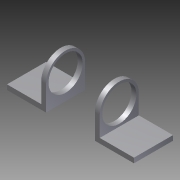
# Autodesk Inventor part: 8 ball arm pivot
Saved by Autodesk Inventor 2012 (Build 160160000, 160)
## iProperties
Created: 2013-10-08
Part Number: 8 ball arm pivot
Material: Default
Document SubType Name: Modeling
Designer: Bryce
Density: 1 g/cm^3
Author: Bryce
Autodesk Inventor part; units mm, degrees
ref_plane "YZ Plane" through (0, 0, 0) normal (1, 0, 0) x (0, 1, 0)
ref_plane "XZ Plane" through (0, 0, 0) normal (0, 1, 0) x (-1, 0, 0)
ref_plane "XY Plane" through (0, 0, 0) normal (0, 0, 1) x (1, 0, 0)
sketch "Sketch1" plane through (0, 0, 0) normal (0, 0, 1) x (1, 0, 0)
  line L0 (0, 0) -> (25.4, 0)
  line L1 (25.4, 0) -> (25.4, 28.575)
  line L2 (25.4, 28.575) -> (22.225, 28.575)
  line L3 (0, 3.175) -> (0, 0)
  line L4 (22.225, 28.575) -> (22.225, 3.175)
  line L5 (22.225, 3.175) -> (0, 3.175)
  line L6 (41.275, 28.575) -> (41.275, 0) construction
  line L7 (82.55, 0) -> (57.15, 0)
  line L8 (57.15, 0) -> (57.15, 28.575)
  line L9 (57.15, 28.575) -> (60.325, 28.575)
  line L10 (82.55, 3.175) -> (82.55, 0)
  line L11 (60.325, 28.575) -> (60.325, 3.175)
  line L12 (60.325, 3.175) -> (82.55, 3.175)
  dimension "d0" = 3.175
  dimension "d1" = 3.175
  dimension "d2" = 25.4
  dimension "d3" = 28.575
  dimension "d4" = 15.875
  constraints: 26 end point, 6 symmetric about line, 2 parallel, 1 horizontal, 1 perpendicular, 1 point on line
  measures "d0" distance between parallel lines of L0 L5
  measures "d1" distance between parallel lines of L1 L4
  measures "d2" distance of L0.start L0.end
  measures "d3" distance of L0.end L1.end
  measures "d4" distance between parallel lines of L6 L1
extrude "Extrusion1" add sketch "Sketch1" along normal blind 25.4
sketch "Sketch2" plane through (60.325, 3.175, 0) normal (1, 0, 0) x (0, 0, -1)
  line L0 (-25.4, 25.4) -> (-25.4, 0) projected
  line L1 (0, 0) -> (-25.4, 0) projected
  line L2 (0, 0) -> (0, 25.4) projected
  line L3 (0, 25.4) -> (-25.4, 25.4) projected
  line L4 (0, -3.175) -> (-25.4, -3.175) projected
  line L5 (-25.4, 0) -> (-25.4, -3.175) projected
  line L6 (0, -3.175) -> (0, 0) projected
  circle A0 centre (-12.7, 12.7) radius 11.1125
  arc A1 (0, 12.7) -> (-25.4, 12.7) centre (-12.7, 12.7) ccw
  dimension "d7" = 22.225
  dimension "d8" = 15.875
  dimension "d9" = 12.7
  constraints: 2 centre point, 2 midpoint, 2 point on circle, 1 tangent
  measures "d7" diameter of A0
  measures "d8" distance from line of L4 A0.centre
  measures "d9" distance from line of L0 A0.centre
extrude "Extrusion2" cut sketch "Sketch2" against normal through all contours L3 A1 L0 | L3 L2 A1 | A0
equation "\"d1\" = d0"
body "Solid1"
